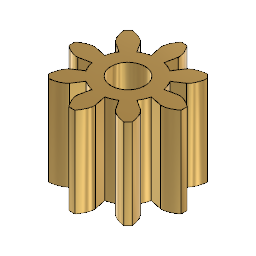
Faulhaber_1717SR006 (Autodesk Fusion 360 archive; units mm, degrees)
design "M0.5 T8 1.5mm Shaft"
description: Spur Gear; Module: 0.500000; Num Teeth: 8; Pressure Angle: 20.000000; Backlash: 0.00 mm
description: Spur Gear; Module: 0.500000; Num Teeth: 10; Pressure Angle: 20.000000; Backlash: 0.00 mm
description: Spur Gear; Module: 0.500000; Num Teeth: 12; Pressure Angle: 20.000000; Backlash: 0.00 mm
Autodesk Fusion 360 part; units mm, degrees
sketch "Sketch1" plane through (0, 0, 0) normal (0, 0, 1) x (1, 0, 0) in component "Spur Gear (8 teeth)"
  circle A0 centre (0, 0) radius 1.3492
  circle A1 centre (0, 0) radius 0.75
  dimension "d7" = 1.5
  measures "d7" diameter of A1
extrude "Extrude1" add sketch "Sketch1" along normal blind 4 makes body 1 in component "Spur Gear (8 teeth)"
sketch "Sketch2" plane through (0, 0, 0) normal (0, 0, 1) x (1, 0, 0) in component "Spur Gear (8 teeth)"
  spline S0 degree 5 poles (1.8376, -0.3941) (1.8394, -0.3945) (1.843, -0.3951) (1.8483, -0.396) (1.8556, -0.3967) (1.8647, -0.3972) (1.8738, -0.3972) (1.8831, -0.397) (1.8923, -0.3967) (1.9016, -0.3963) (1.9109, -0.3958) (1.9202, -0.3952) (1.9295, -0.3944) (1.9389, -0.3934) (1.9483, -0.3922) (1.9577, -0.3909) (1.9671, -0.3894) (1.9766, -0.3877) (1.986, -0.386) (1.9955, -0.3841) (2.005, -0.3821) (2.0145, -0.38) (2.024, -0.3778) (2.0335, -0.3755) (2.043, -0.373) (2.0526, -0.3704) (2.0621, -0.3677) (2.0717, -0.3649) (2.0812, -0.362) (2.0908, -0.359) (2.1003, -0.3558) (2.1099, -0.3526) (2.1195, -0.3492) (2.129, -0.3458) (2.1386, -0.3422) (2.1482, -0.3385) (2.1577, -0.3347) (2.1673, -0.3309) (2.1769, -0.3269) (2.1864, -0.3228) (2.196, -0.3186) (2.2056, -0.3144) (2.2151, -0.31) (2.2246, -0.3055) (2.2342, -0.3009) (2.2437, -0.2963) (2.2532, -0.2915) (2.2628, -0.2866) (2.2723, -0.2817) (2.2818, -0.2766) (2.2913, -0.2715) (2.3007, -0.2663) (2.3102, -0.2609) (2.3197, -0.2555) (2.3291, -0.25) (2.3385, -0.2444) (2.3479, -0.2387) (2.3574, -0.2329) (2.3667, -0.227) (2.3761, -0.221) (2.3855, -0.2149) (2.3948, -0.2088) (2.4041, -0.2025) (2.4134, -0.1962) (2.4227, -0.1898) (2.432, -0.1833) (2.4413, -0.1767) (2.4505, -0.17) (2.4597, -0.1632) (2.4689, -0.1564) (2.4781, -0.1494) (2.4854, -0.1438) (2.4909, -0.1395) (2.4945, -0.1367) (2.4963, -0.1352) knots 0 0 0 0 0 0 0.01428571 0.02857143 0.04285714 0.05714286 0.07142857 0.08571429 0.1 0.11428571 0.12857143 0.14285714 0.15714286 0.17142857 0.18571429 0.2 0.21428571 0.22857143 0.24285714 0.25714286 0.27142857 0.28571429 0.3 0.31428571 0.32857143 0.34285714 0.35714286 0.37142857 0.38571429 0.4 0.41428571 0.42857143 0.44285714 0.45714286 0.47142857 0.48571429 0.5 0.51428571 0.52857143 0.54285714 0.55714286 0.57142857 0.58571429 0.6 0.61428571 0.62857143 0.64285714 0.65714286 0.67142857 0.68571429 0.7 0.71428571 0.72857143 0.74285714 0.75714286 0.77142857 0.78571429 0.8 0.81428571 0.82857143 0.84285714 0.85714286 0.87142857 0.88571429 0.9 0.91428571 0.92857143 0.94285714 0.95714286 0.97142857 0.98571429 1 1 1 1 1 1
  spline S1 degree 5 poles (1.8376, 0.3941) (1.8394, 0.3945) (1.843, 0.3951) (1.8483, 0.396) (1.8556, 0.3967) (1.8647, 0.3972) (1.8738, 0.3972) (1.8831, 0.397) (1.8923, 0.3967) (1.9016, 0.3963) (1.9109, 0.3958) (1.9202, 0.3952) (1.9295, 0.3944) (1.9389, 0.3934) (1.9483, 0.3922) (1.9577, 0.3909) (1.9671, 0.3894) (1.9766, 0.3877) (1.986, 0.386) (1.9955, 0.3841) (2.005, 0.3821) (2.0145, 0.38) (2.024, 0.3778) (2.0335, 0.3755) (2.043, 0.373) (2.0526, 0.3704) (2.0621, 0.3677) (2.0717, 0.3649) (2.0812, 0.362) (2.0908, 0.359) (2.1003, 0.3558) (2.1099, 0.3526) (2.1195, 0.3492) (2.129, 0.3458) (2.1386, 0.3422) (2.1482, 0.3385) (2.1577, 0.3347) (2.1673, 0.3309) (2.1769, 0.3269) (2.1864, 0.3228) (2.196, 0.3186) (2.2056, 0.3144) (2.2151, 0.31) (2.2246, 0.3055) (2.2342, 0.3009) (2.2437, 0.2963) (2.2532, 0.2915) (2.2628, 0.2866) (2.2723, 0.2817) (2.2818, 0.2766) (2.2913, 0.2715) (2.3007, 0.2663) (2.3102, 0.2609) (2.3197, 0.2555) (2.3291, 0.25) (2.3385, 0.2444) (2.3479, 0.2387) (2.3574, 0.2329) (2.3667, 0.227) (2.3761, 0.221) (2.3855, 0.2149) (2.3948, 0.2088) (2.4041, 0.2025) (2.4134, 0.1962) (2.4227, 0.1898) (2.432, 0.1833) (2.4413, 0.1767) (2.4505, 0.17) (2.4597, 0.1632) (2.4689, 0.1564) (2.4781, 0.1494) (2.4854, 0.1438) (2.4909, 0.1395) (2.4945, 0.1367) (2.4963, 0.1352) knots 0 0 0 0 0 0 0.01428571 0.02857143 0.04285714 0.05714286 0.07142857 0.08571429 0.1 0.11428571 0.12857143 0.14285714 0.15714286 0.17142857 0.18571429 0.2 0.21428571 0.22857143 0.24285714 0.25714286 0.27142857 0.28571429 0.3 0.31428571 0.32857143 0.34285714 0.35714286 0.37142857 0.38571429 0.4 0.41428571 0.42857143 0.44285714 0.45714286 0.47142857 0.48571429 0.5 0.51428571 0.52857143 0.54285714 0.55714286 0.57142857 0.58571429 0.6 0.61428571 0.62857143 0.64285714 0.65714286 0.67142857 0.68571429 0.7 0.71428571 0.72857143 0.74285714 0.75714286 0.77142857 0.78571429 0.8 0.81428571 0.82857143 0.84285714 0.85714286 0.87142857 0.88571429 0.9 0.91428571 0.92857143 0.94285714 0.95714286 0.97142857 0.98571429 1 1 1 1 1 1
  arc A0 (2.4963, -0.1352) -> (2.4963, 0.1352) centre (0, 0) ccw
  line L0 (1.3094, -0.2829) -> (1.8376, -0.3941)
  line L1 (1.3094, 0.2829) -> (1.8376, 0.3941)
  line L2 (1.3094, -0.2829) -> (1.3094, 0.2829)
extrude "Extrude2" add sketch "Sketch2" along normal blind 4 bodies 1 in component "Spur Gear (8 teeth)"
pattern_circular "C-Pattern1" count 8 over 360 about axis through (0, 0, 0) along (0, 0, 1) of "Extrude2" in component "Spur Gear (8 teeth)"
sketch "Sketch3" plane through (0, 0, 0) normal (0, 0, 1) x (1, 0, 0) in component "Spur Gear (8 teeth)"
  circle A0 centre (0, 0) radius 2 construction
sketch "Sketch1 (2)" plane through (0, 0, 0) normal (0, 0, 1) x (1, 0, 0) in component "Spur Gear (10 teeth)"
  circle A0 centre (0, 0) radius 1.8492
  circle A1 centre (0, 0) radius 0.75
extrude "Extrude1'" add sketch "Sketch1 (2)" along normal blind 4 separate body makes body 2 in component "Spur Gear (10 teeth)"
sketch "Sketch2 (2)" plane through (0, 0, 0) normal (0, 0, 1) x (1, 0, 0) in component "Spur Gear (10 teeth)"
  spline S0 degree 5 poles (2.3146, -0.402) (2.3164, -0.4024) (2.3202, -0.4029) (2.3258, -0.4036) (2.3334, -0.4042) (2.3429, -0.4044) (2.3525, -0.4042) (2.3621, -0.4039) (2.3717, -0.4034) (2.3814, -0.4028) (2.3911, -0.4021) (2.4007, -0.4013) (2.4104, -0.4003) (2.4202, -0.3992) (2.4299, -0.3979) (2.4396, -0.3964) (2.4494, -0.3947) (2.4592, -0.393) (2.469, -0.3911) (2.4788, -0.3892) (2.4886, -0.3871) (2.4984, -0.3849) (2.5082, -0.3826) (2.518, -0.3802) (2.5279, -0.3777) (2.5377, -0.3751) (2.5476, -0.3723) (2.5574, -0.3695) (2.5673, -0.3665) (2.5771, -0.3634) (2.587, -0.3603) (2.5968, -0.357) (2.6067, -0.3537) (2.6166, -0.3503) (2.6264, -0.3467) (2.6363, -0.3431) (2.6462, -0.3393) (2.656, -0.3355) (2.6659, -0.3316) (2.6757, -0.3276) (2.6856, -0.3235) (2.6954, -0.3193) (2.7053, -0.315) (2.7151, -0.3106) (2.7249, -0.3061) (2.7348, -0.3016) (2.7446, -0.2969) (2.7544, -0.2922) (2.7642, -0.2874) (2.774, -0.2825) (2.7838, -0.2775) (2.7936, -0.2724) (2.8034, -0.2673) (2.8131, -0.262) (2.8229, -0.2567) (2.8327, -0.2513) (2.8424, -0.2458) (2.8521, -0.2402) (2.8618, -0.2346) (2.8715, -0.2288) (2.8812, -0.223) (2.8909, -0.2171) (2.9006, -0.2111) (2.9102, -0.2051) (2.9199, -0.1989) (2.9295, -0.1927) (2.9391, -0.1864) (2.9487, -0.18) (2.9583, -0.1735) (2.9678, -0.167) (2.9774, -0.1604) (2.985, -0.155) (2.9907, -0.151) (2.9945, -0.1482) (2.9964, -0.1469) knots 0 0 0 0 0 0 0.01428571 0.02857143 0.04285714 0.05714286 0.07142857 0.08571429 0.1 0.11428571 0.12857143 0.14285714 0.15714286 0.17142857 0.18571429 0.2 0.21428571 0.22857143 0.24285714 0.25714286 0.27142857 0.28571429 0.3 0.31428571 0.32857143 0.34285714 0.35714286 0.37142857 0.38571429 0.4 0.41428571 0.42857143 0.44285714 0.45714286 0.47142857 0.48571429 0.5 0.51428571 0.52857143 0.54285714 0.55714286 0.57142857 0.58571429 0.6 0.61428571 0.62857143 0.64285714 0.65714286 0.67142857 0.68571429 0.7 0.71428571 0.72857143 0.74285714 0.75714286 0.77142857 0.78571429 0.8 0.81428571 0.82857143 0.84285714 0.85714286 0.87142857 0.88571429 0.9 0.91428571 0.92857143 0.94285714 0.95714286 0.97142857 0.98571429 1 1 1 1 1 1
  spline S1 degree 5 poles (2.3146, 0.402) (2.3164, 0.4024) (2.3202, 0.4029) (2.3258, 0.4036) (2.3334, 0.4042) (2.3429, 0.4044) (2.3525, 0.4042) (2.3621, 0.4039) (2.3717, 0.4034) (2.3814, 0.4028) (2.3911, 0.4021) (2.4007, 0.4013) (2.4104, 0.4003) (2.4202, 0.3992) (2.4299, 0.3979) (2.4396, 0.3964) (2.4494, 0.3947) (2.4592, 0.393) (2.469, 0.3911) (2.4788, 0.3892) (2.4886, 0.3871) (2.4984, 0.3849) (2.5082, 0.3826) (2.518, 0.3802) (2.5279, 0.3777) (2.5377, 0.3751) (2.5476, 0.3723) (2.5574, 0.3695) (2.5673, 0.3665) (2.5771, 0.3634) (2.587, 0.3603) (2.5968, 0.357) (2.6067, 0.3537) (2.6166, 0.3503) (2.6264, 0.3467) (2.6363, 0.3431) (2.6462, 0.3393) (2.656, 0.3355) (2.6659, 0.3316) (2.6757, 0.3276) (2.6856, 0.3235) (2.6954, 0.3193) (2.7053, 0.315) (2.7151, 0.3106) (2.7249, 0.3061) (2.7348, 0.3016) (2.7446, 0.2969) (2.7544, 0.2922) (2.7642, 0.2874) (2.774, 0.2825) (2.7838, 0.2775) (2.7936, 0.2724) (2.8034, 0.2673) (2.8131, 0.262) (2.8229, 0.2567) (2.8327, 0.2513) (2.8424, 0.2458) (2.8521, 0.2402) (2.8618, 0.2346) (2.8715, 0.2288) (2.8812, 0.223) (2.8909, 0.2171) (2.9006, 0.2111) (2.9102, 0.2051) (2.9199, 0.1989) (2.9295, 0.1927) (2.9391, 0.1864) (2.9487, 0.18) (2.9583, 0.1735) (2.9678, 0.167) (2.9774, 0.1604) (2.985, 0.155) (2.9907, 0.151) (2.9945, 0.1482) (2.9964, 0.1469) knots 0 0 0 0 0 0 0.01428571 0.02857143 0.04285714 0.05714286 0.07142857 0.08571429 0.1 0.11428571 0.12857143 0.14285714 0.15714286 0.17142857 0.18571429 0.2 0.21428571 0.22857143 0.24285714 0.25714286 0.27142857 0.28571429 0.3 0.31428571 0.32857143 0.34285714 0.35714286 0.37142857 0.38571429 0.4 0.41428571 0.42857143 0.44285714 0.45714286 0.47142857 0.48571429 0.5 0.51428571 0.52857143 0.54285714 0.55714286 0.57142857 0.58571429 0.6 0.61428571 0.62857143 0.64285714 0.65714286 0.67142857 0.68571429 0.7 0.71428571 0.72857143 0.74285714 0.75714286 0.77142857 0.78571429 0.8 0.81428571 0.82857143 0.84285714 0.85714286 0.87142857 0.88571429 0.9 0.91428571 0.92857143 0.94285714 0.95714286 0.97142857 0.98571429 1 1 1 1 1 1
  arc A0 (2.9964, -0.1469) -> (2.9964, 0.1469) centre (0, 0) ccw
  line L0 (1.8121, -0.3165) -> (2.3146, -0.402)
  line L1 (1.8121, 0.3165) -> (2.3146, 0.402)
  line L2 (1.8121, -0.3165) -> (1.8121, 0.3165)
extrude "Extrude2'" add sketch "Sketch2 (2)" along normal blind 4 bodies 2 in component "Spur Gear (10 teeth)"
pattern_circular "C-Pattern1'" count 10 over 360 about axis through (0, 0, 0) along (0, 0, 1) of "Extrude2'" in component "Spur Gear (10 teeth)"
sketch "Sketch3 (2)" plane through (0, 0, 0) normal (0, 0, 1) x (1, 0, 0) in component "Spur Gear (10 teeth)"
  circle A0 centre (0, 0) radius 2.5 construction
sketch "Sketch1 (3)" plane through (0, 0, 0) normal (0, 0, 1) x (1, 0, 0) in component "Spur Gear (12 teeth)"
  circle A0 centre (0, 0) radius 2.3492
  circle A1 centre (0, 0) radius 0.75
extrude "Extrude1''" add sketch "Sketch1 (3)" along normal blind 4 separate body makes body 3 in component "Spur Gear (12 teeth)"
sketch "Sketch2 (3)" plane through (0, 0, 0) normal (0, 0, 1) x (1, 0, 0) in component "Spur Gear (12 teeth)"
  spline S0 degree 5 poles (2.7892, -0.4096) (2.7911, -0.4099) (2.7951, -0.4104) (2.801, -0.4109) (2.8089, -0.4114) (2.8188, -0.4114) (2.8288, -0.4111) (2.8388, -0.4106) (2.8488, -0.41) (2.8589, -0.4093) (2.8689, -0.4084) (2.879, -0.4075) (2.8891, -0.4064) (2.8992, -0.4052) (2.9093, -0.4038) (2.9194, -0.4022) (2.9296, -0.4005) (2.9397, -0.3986) (2.9499, -0.3967) (2.96, -0.3946) (2.9702, -0.3925) (2.9804, -0.3902) (2.9905, -0.3879) (3.0007, -0.3854) (3.0109, -0.3828) (3.0211, -0.3801) (3.0313, -0.3773) (3.0415, -0.3744) (3.0517, -0.3715) (3.0619, -0.3684) (3.0721, -0.3652) (3.0823, -0.3619) (3.0925, -0.3586) (3.1027, -0.3551) (3.1129, -0.3515) (3.1231, -0.3479) (3.1333, -0.3442) (3.1435, -0.3403) (3.1537, -0.3364) (3.1639, -0.3324) (3.1741, -0.3284) (3.1843, -0.3242) (3.1945, -0.3199) (3.2047, -0.3156) (3.2149, -0.3112) (3.225, -0.3067) (3.2352, -0.3021) (3.2454, -0.2974) (3.2555, -0.2927) (3.2657, -0.2878) (3.2758, -0.2829) (3.286, -0.2779) (3.2961, -0.2728) (3.3062, -0.2677) (3.3163, -0.2625) (3.3264, -0.2571) (3.3365, -0.2518) (3.3466, -0.2463) (3.3567, -0.2407) (3.3668, -0.2351) (3.3768, -0.2294) (3.3869, -0.2236) (3.3969, -0.2178) (3.4069, -0.2119) (3.4169, -0.2059) (3.4269, -0.1998) (3.4369, -0.1936) (3.4469, -0.1874) (3.4569, -0.1811) (3.4668, -0.1747) (3.4767, -0.1683) (3.4847, -0.1631) (3.4906, -0.1591) (3.4946, -0.1565) (3.4966, -0.1552) knots 0 0 0 0 0 0 0.01428571 0.02857143 0.04285714 0.05714286 0.07142857 0.08571429 0.1 0.11428571 0.12857143 0.14285714 0.15714286 0.17142857 0.18571429 0.2 0.21428571 0.22857143 0.24285714 0.25714286 0.27142857 0.28571429 0.3 0.31428571 0.32857143 0.34285714 0.35714286 0.37142857 0.38571429 0.4 0.41428571 0.42857143 0.44285714 0.45714286 0.47142857 0.48571429 0.5 0.51428571 0.52857143 0.54285714 0.55714286 0.57142857 0.58571429 0.6 0.61428571 0.62857143 0.64285714 0.65714286 0.67142857 0.68571429 0.7 0.71428571 0.72857143 0.74285714 0.75714286 0.77142857 0.78571429 0.8 0.81428571 0.82857143 0.84285714 0.85714286 0.87142857 0.88571429 0.9 0.91428571 0.92857143 0.94285714 0.95714286 0.97142857 0.98571429 1 1 1 1 1 1
  spline S1 degree 5 poles (2.7892, 0.4096) (2.7911, 0.4099) (2.7951, 0.4104) (2.801, 0.4109) (2.8089, 0.4114) (2.8188, 0.4114) (2.8288, 0.4111) (2.8388, 0.4106) (2.8488, 0.41) (2.8589, 0.4093) (2.8689, 0.4084) (2.879, 0.4075) (2.8891, 0.4064) (2.8992, 0.4052) (2.9093, 0.4038) (2.9194, 0.4022) (2.9296, 0.4005) (2.9397, 0.3986) (2.9499, 0.3967) (2.96, 0.3946) (2.9702, 0.3925) (2.9804, 0.3902) (2.9905, 0.3879) (3.0007, 0.3854) (3.0109, 0.3828) (3.0211, 0.3801) (3.0313, 0.3773) (3.0415, 0.3744) (3.0517, 0.3715) (3.0619, 0.3684) (3.0721, 0.3652) (3.0823, 0.3619) (3.0925, 0.3586) (3.1027, 0.3551) (3.1129, 0.3515) (3.1231, 0.3479) (3.1333, 0.3442) (3.1435, 0.3403) (3.1537, 0.3364) (3.1639, 0.3324) (3.1741, 0.3284) (3.1843, 0.3242) (3.1945, 0.3199) (3.2047, 0.3156) (3.2149, 0.3112) (3.225, 0.3067) (3.2352, 0.3021) (3.2454, 0.2974) (3.2555, 0.2927) (3.2657, 0.2878) (3.2758, 0.2829) (3.286, 0.2779) (3.2961, 0.2728) (3.3062, 0.2677) (3.3163, 0.2625) (3.3264, 0.2571) (3.3365, 0.2518) (3.3466, 0.2463) (3.3567, 0.2407) (3.3668, 0.2351) (3.3768, 0.2294) (3.3869, 0.2236) (3.3969, 0.2178) (3.4069, 0.2119) (3.4169, 0.2059) (3.4269, 0.1998) (3.4369, 0.1936) (3.4469, 0.1874) (3.4569, 0.1811) (3.4668, 0.1747) (3.4767, 0.1683) (3.4847, 0.1631) (3.4906, 0.1591) (3.4946, 0.1565) (3.4966, 0.1552) knots 0 0 0 0 0 0 0.01428571 0.02857143 0.04285714 0.05714286 0.07142857 0.08571429 0.1 0.11428571 0.12857143 0.14285714 0.15714286 0.17142857 0.18571429 0.2 0.21428571 0.22857143 0.24285714 0.25714286 0.27142857 0.28571429 0.3 0.31428571 0.32857143 0.34285714 0.35714286 0.37142857 0.38571429 0.4 0.41428571 0.42857143 0.44285714 0.45714286 0.47142857 0.48571429 0.5 0.51428571 0.52857143 0.54285714 0.55714286 0.57142857 0.58571429 0.6 0.61428571 0.62857143 0.64285714 0.65714286 0.67142857 0.68571429 0.7 0.71428571 0.72857143 0.74285714 0.75714286 0.77142857 0.78571429 0.8 0.81428571 0.82857143 0.84285714 0.85714286 0.87142857 0.88571429 0.9 0.91428571 0.92857143 0.94285714 0.95714286 0.97142857 0.98571429 1 1 1 1 1 1
  arc A0 (3.4966, -0.1552) -> (3.4966, 0.1552) centre (0, 0) ccw
  line L0 (2.3144, -0.3413) -> (2.7892, -0.4096)
  line L1 (2.3144, 0.3413) -> (2.7892, 0.4096)
  line L2 (2.3144, -0.3413) -> (2.3144, 0.3413)
extrude "Extrude2''" add sketch "Sketch2 (3)" along normal blind 4 bodies 3 in component "Spur Gear (12 teeth)"
pattern_circular "C-Pattern1''" count 12 over 360 about axis through (0, 0, 0) along (0, 0, 1) of "Extrude2''" in component "Spur Gear (12 teeth)"
sketch "Sketch3 (3)" plane through (0, 0, 0) normal (0, 0, 1) x (1, 0, 0) in component "Spur Gear (12 teeth)"
  circle A0 centre (0, 0) radius 3 construction
component "Spur Gear (8 teeth)" placed x (1, 0, 0) y (0, 1, 0) z (0, 0, 1) at (0, 0, 0)
component "Spur Gear (10 teeth)" placed x (1, 0, 0) y (0, 1, 0) z (0, 0, 1) at (0, 0, 0)
component "Spur Gear (12 teeth)" placed x (1, 0, 0) y (0, 1, 0) z (0, 0, 1) at (0, 0, 0)
named bodies: "T8"
